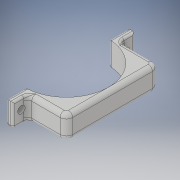
# Autodesk Inventor part: 35mm petri dish stage_heating2
Saved by Autodesk Inventor 2018 (Build 220112000, 112)
## iProperties
Created: 2018-07-03
Part Number: 35mm petri dish stage_heating2
Material: Generic
Document SubType Name: Modeling
Designer: Iek Man Lei
Density: 1 g/cm^3
Appearance: Default
Author: Iek Man Lei
Autodesk Inventor part; units mm, degrees
ref_plane "YZ Plane" through (0, 0, 0) normal (1, 0, 0) x (0, 1, 0)
ref_plane "XZ Plane" through (0, 0, 0) normal (0, 1, 0) x (-1, 0, 0)
ref_plane "XY Plane" through (0, 0, 0) normal (0, 0, 1) x (1, 0, 0)
sketch "Sketch1" plane through (0, 0, 0) normal (0, 1, 0) x (-1, 0, 0)
  line L0 (29.6667, 24) -> (-23.3333, 24)
  line L1 (-23.3333, 24) -> (-23.3333, -20)
  line L2 (-23.3333, -20) -> (29.6667, -20)
  line L3 (29.6667, -20) -> (29.6667, 24)
  point P0 (0, 0)
  dimension "d0" = 44
  dimension "d1" = 53
  constraints: 8 end point, 2 parallel, 1 horizontal, 1 perpendicular
  measures "d0" distance of L0.end L1.end
  measures "d1" distance of L1.end L2.end
extrude "Extrusion1" add sketch "Sketch1" along normal blind 11
sketch "Sketch2" plane through (0, 11, 0) normal (0, 1, 0) x (1, 0, 0)
  circle A0 centre (1.3333, -2) radius 20
  line L0 (23.3333, -24) -> (23.3333, 20) projected
  line L1 (23.3333, 20) -> (-29.6667, 20) projected
  point P0 (0, 0)
  dimension "d4" = 40
  dimension "d5" = 22
  dimension "d27" = 22
  constraints: 1 centre point
  measures "d4" diameter of A0
  measures "d5" distance from line of L0 A0.centre
  measures "d27" distance from line of L1 A0.centre
extrude "Extrusion2" cut sketch "Sketch2" against normal blind 38
sketch "Sketch4" plane through (0, 11, 0) normal (0, 1, 0) x (1, 0, 0)
  line L0 (-29.6667, -24) -> (-24.6667, -24)
  line L1 (-24.6667, -24) -> (-24.6667, 20)
  line L2 (-24.6667, 20) -> (-29.6667, 20)
  line L3 (-29.6667, 20) -> (-29.6667, -24)
  line L4 (-29.6667, 20) -> (-29.6667, -24) projected
  line L5 (23.3333, 20) -> (-29.6667, 20) projected
  point P0 (0, 0)
  dimension "d12" = 5
  dimension "d13" = 44
  constraints: 8 end point, 2 collinear, 2 parallel, 1 horizontal, 1 perpendicular
  measures "d12" distance of L1.end L2.end
  measures "d13" distance of L0.end L1.end
extrude "Extrusion3" add sketch "Sketch4" against normal blind 10
fillet "Fillet1" radius 3 2 edges at (23.3333, 5.5, -20) (23.3333, 5.5, 24)
fillet "Fillet4" radius 1 1 edges at (-29.6667, 0, 2)
sketch "Sketch9" plane through (0, 11, 0) normal (0, 1, 0) x (1, 0, 0)
  line L0 (20.3333, 20) -> (-28.6667, 20) projected
  line L1 (-29.6667, -24) -> (-23.6667, -24)
  line L2 (-23.6667, -24) -> (-23.6667, 20)
  line L3 (-23.6667, 20) -> (-29.6667, 20)
  line L4 (-29.6667, 20) -> (-29.6667, -24)
  line L5 (-29.6667, 20) -> (-29.6667, -24) projected
  point P0 (0, 0)
  dimension "d45" = 6
  dimension "d63" = 44
  constraints: 8 end point, 2 parallel, 1 collinear, 1 horizontal, 1 perpendicular, 1 point on line
  measures "d45" distance of L3.end L2.end
  measures "d63" distance of L3.end L1.start
extrude "Extrusion8" add sketch "Sketch9" along normal blind 13
sketch "Sketch10" plane through (-23.6667, 11, 24) normal (1, 0, 0) x (0, 0, -1)
  circle A0 centre (14, 7) radius 1.75
  circle A1 centre (30, 7) radius 1.75
  line L0 (44, 0) -> (44, 13) projected
  line L1 (0, 0) -> (0, 13) projected
  line L2 (0, 13) -> (44, 13) projected
  circle A2 centre (22, 7) radius 1.75
  point P0 (24, -11)
  dimension "d48" = 3.5
  dimension "d49" = 3.5
  dimension "d50" = 16
  dimension "d51" = 14
  dimension "d53" = 6
  dimension "d62" = 14
  dimension "d64" = 3.5
  dimension "d65" = 8
  constraints: 3 centre point, 2 horizontal alignment
  measures "d48" diameter of A0
  measures "d49" diameter of A1
  measures "d50" distance of A1.centre A0.centre
  measures "d51" distance from line of A1.centre L0
  measures "d53" distance from line of A1.centre L2
  measures "d62" distance from line of L1 A0.centre
  measures "d64" diameter of A2
  measures "d65" distance of A0.centre A2.centre
extrude "Extrusion9" cut sketch "Sketch10" against normal blind 10
sketch "Sketch11" plane through (-23.6667, 11, 24) normal (1, 0, 0) x (0, 0, -1)
  line L0 (0, 0) -> (0, 13) projected
  circle A0 centre (0, 13) radius 10
  line L1 (44, -10) -> (44, 13) projected
  circle A1 centre (44, 13) radius 10
  point P0 (24, -11)
  dimension "d56" = 20
  dimension "d57" = 20
  constraints: 2 centre point
  measures "d56" diameter of A0
  measures "d57" diameter of A1
extrude "Extrusion10" cut sketch "Sketch11" against normal blind 10
fillet "Fillet5" radius 3 1 edges at (-23.6667, 11, 2)
sketch "Sketch12" plane through (0, 0, 0) normal (0, -1, 0) x (1, 0, 0)
  circle A0 centre (18.3333, 19) radius 1.75
  line L0 (20.3333, 24) -> (-27.6667, 24) projected
  line L1 (23.3333, -17) -> (23.3333, 21) projected
  circle A1 centre (-15.6667, 19) radius 1.75
  circle A2 centre (18.3333, -15) radius 1.75
  circle A3 centre (-15.6667, -15) radius 1.75
  point P0 (0, 0)
  dimension "d66" = 3.5
  dimension "d67" = 5
  dimension "d68" = 5
  dimension "d71" = 34
  dimension "d74" = 34
  constraints: 4 centre point, 1 horizontal, 1 vertical, 6 other
  measures "d66" diameter of A0
  measures "d67" distance from line of L0 A0.centre
  measures "d68" distance from line of A0.centre L1
  measures "d71" distance of A0.centre A1.centre
  measures "d74" distance of A0.centre A2.centre
extrude "Extrusion11" cut sketch "Sketch12" against normal blind 2.4
sketch "Sketch13" plane through (0, 11, 0) normal (0, 1, 0) x (1, 0, 0)
  line L0 (-30.1625, 22.225) -> (1.8333, 22.225)
  line L1 (1.8333, 22.225) -> (1.8333, -31.75)
  line L2 (1.8333, -31.75) -> (-30.1625, -31.75)
  line L3 (-30.1625, -31.75) -> (-30.1625, 22.225)
  line L4 (23.3333, -21) -> (23.3333, 17) projected
  point P0 (0, 0)
  dimension "d79" = 21.5
  constraints: 8 end point, 2 parallel, 1 horizontal, 1 perpendicular
  measures "d79" distance between parallel lines of L4 L1
extrude "Extrusion12" cut sketch "Sketch13" against normal blind 11 and the other way blind 15
sketch "Sketch14" plane through (20.3333, 0, -20) normal (0, 0, -1) x (-1, 0, 0)
  line L0 (18.5, 11) -> (18.5, 0) projected
  line L1 (0, 0) -> (49, 0) projected
  line L2 (18.5, 11) -> (15.5, 11)
  line L3 (15.5, 11) -> (15.5, 0)
  line L4 (15.5, 0) -> (18.5, 0)
  line L5 (18.5, 0) -> (18.5, 11)
  point P0 (20.3333, 0)
  point P1 (18.5, 1)
  dimension "d84" = 3
  constraints: 8 end point, 2 parallel, 1 horizontal, 1 perpendicular, 1 point on line
  measures "d84" distance of L4.end L3.end
extrude "Extrusion13" add sketch "Sketch14" along normal blind 7
sketch "Sketch15" plane through (20.3333, 0, 24) normal (0, 0, 1) x (1, 0, 0)
  line L0 (-18.5, 11) -> (-18.5, 0) projected
  line L1 (-15.5, 11) -> (-15.5, 0) projected
  line L2 (-18.5, 11) -> (-15.5, 11)
  line L3 (-15.5, 11) -> (-15.5, 0)
  line L4 (-15.5, 0) -> (-18.5, 0)
  line L5 (-18.5, 0) -> (-18.5, 11)
  point P0 (-20.3333, 0)
  point P1 (-18.5, 1)
  dimension "d101" = 3
  constraints: 8 end point, 2 parallel, 1 horizontal, 1 perpendicular
  measures "d101" distance of L1.end L4.end
extrude "Extrusion14" add sketch "Sketch15" along normal blind 7
sketch "Sketch16" plane through (1.8333, 0, -17.9937) normal (-1, 0, 0) x (0, 0, 1)
  circle A0 centre (-5.0063, 5) radius 1.7
  circle A1 centre (44.9937, 6) radius 1.7
  line L0 (-9.0063, 0) -> (-9.0063, 11) projected
  line L1 (0, 0) -> (-9.0063, 0) projected
  line L2 (39.9875, 11) -> (48.9937, 11) projected
  line L3 (48.9937, 11) -> (48.9937, 0) projected
  point P0 (17.9937, 0)
  point P1 (-2.0063, 0)
  dimension "d89" = 3.4
  dimension "d90" = 3.4
  dimension "d91" = 4
  dimension "d92" = 5
  dimension "d93" = 5
  dimension "d94" = 4
  constraints: 2 centre point
  measures "d89" diameter of A0
  measures "d90" diameter of A1
  measures "d91" distance from line of A0.centre L0
  measures "d92" distance from line of L1 A0.centre
  measures "d93" distance from line of A1.centre L2
  measures "d94" distance from line of L3 A1.centre
extrude "Extrusion15" cut sketch "Sketch16" against normal blind 7
fillet "Fillet7" radius 2 10 edges at (22.4547, 0, -19.1213) (23.3333, 0, 2) (22.4547, 0, 23.1213) (12.5833, 0, 24) (12.5833, 0, -20) (22.4547, 11, -19.1213) (23.3333, 11, 2) (22.4547, 11, 23.1213) (12.5833, 11, 24) (12.5833, 11, -20)
fillet "Fillet8" radius 2 6 edges at (4.8333, 10.4142, -19.4142) (4.8333, 0.5858, -19.4142) (4.8333, 5.5, -20) (4.8333, 0.5858, 23.4142) (4.8333, 10.4142, 23.4142) (4.8333, 5.5, 24)
fillet "Fillet9" radius 1 6 edges at (5.4888, 0, -19.5321) (4.8333, 0, -24.2321) (4.8333, 5.5, -27) (5.4888, 11, -19.5321) (4.8333, 11, -24.2321) (3.3333, 0, 31)
fillet "Fillet10" radius 1 15 edges at (4.8333, 0.2929, 30.7071) (4.8333, 0, 27.7321) (5.4888, 0, 23.5321) (4.8333, 6, 31) (1.8333, 0.2929, 30.7071) (1.8333, 0, 25.9969) (1.8333, 6, 31) (5.4888, 11, 23.5321) (4.8333, 11, 28.2321) (1.8333, 11, 26.4969) (1.8333, 11, -22.4969) (1.8333, 5.5, -27) (1.8333, 0, -22.4969) (1.8333, 5.5, 21.9937) (1.8333, 5.5, -17.9937)
body "Solid1"
